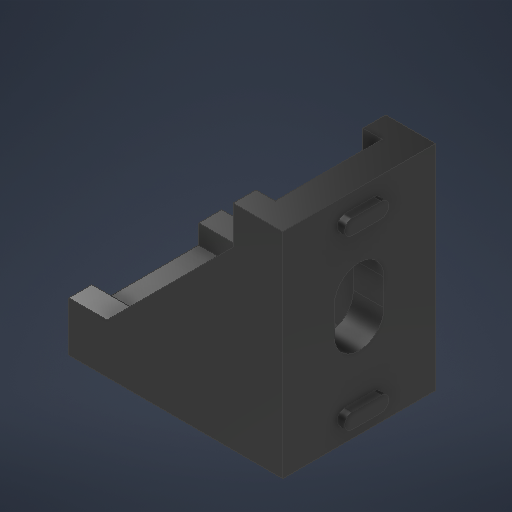
# Autodesk Inventor part: CORNER2028
Saved by Autodesk Inventor 2026.2 (Build 302298010, 298A)
## iProperties
Created: 2026-04-15
Part Number: CORNER2028
Material: Generic
Document SubType Name: Modeling
Designer: grego
Density: 1 g/cm^3
Appearance: Default
Author: grego
Autodesk Inventor part; units mm, degrees
ref_plane "YZ Plane" through (0, 0, 0) normal (1, 0, 0) x (0, 1, 0)
ref_plane "XZ Plane" through (0, 0, 0) normal (0, 1, 0) x (-1, 0, 0)
ref_plane "XY Plane" through (0, 0, 0) normal (0, 0, 1) x (1, 0, 0)
sketch "Sketch1" plane through (0, 0, 0) normal (0, 1, 0) x (-1, 0, 0)
  line L0 (0, 0) -> (28, 0)
  line L1 (28, 0) -> (28, -20)
  line L2 (28, -20) -> (0, -20)
  line L3 (0, -20) -> (0, 0)
  dimension "d0" = 28
  dimension "d1" = 20
  constraints: 8 end point, 2 parallel, 1 horizontal, 1 perpendicular
  measures "d0" distance of L1.end L2.end
  measures "d1" distance of L0.end L1.end
extrude "Extrusion1" add sketch "Sketch1" along normal blind 4
sketch "Sketch2" plane through (0, 4, 0) normal (0, 1, 0) x (1, 0, 0)
  line L0 (0, 20) -> (-28, 20) projected
  line L1 (-28, 20) -> (-28, 0) projected
  line L2 (-28, 0) -> (0, 0) projected
  line L3 (0, 0) -> (0, 20) projected
  line L4 (0, 0) -> (-4, 0)
  line L5 (-4, 0) -> (-4, 20)
  line L6 (-4, 20) -> (0, 20)
  line L7 (0, 20) -> (0, 0)
  dimension "d4" = 4
  constraints: 8 end point, 2 parallel, 1 horizontal, 1 perpendicular, 1 point on line
  measures "d4" distance of L5.end L6.end
extrude "Extrusion2" add sketch "Sketch2" along normal blind 24 contours L3 L2 L5 L0
sketch "Sketch3" plane through (-4, 4, -20) normal (-1, 0, 0) x (0, 0, 1)
  line L0 (20, -4) -> (0, -4) projected
  line L1 (0, -4) -> (0, 24) projected
  line L2 (20, 24) -> (0, 24) projected
  line L3 (20, -4) -> (20, 24) projected
  line L4 (0, -4) -> (0, 24) projected
  line L5 (10, 15.5) -> (10, 15.5)
  line L6 (13.25, 12.25) -> (13.25, 8.75)
  line L7 (10, 5.5) -> (10, 5.5)
  line L8 (6.75, 8.75) -> (6.75, 12.25)
  line L9 (6.75, 15.5) -> (13.25, 5.5) construction
  line L10 (13.25, 15.5) -> (6.75, 5.5) construction
  arc A0 (10, 5.5) -> (13.25, 8.75) centre (10, 8.75) ccw
  arc A1 (6.75, 8.75) -> (10, 5.5) centre (10, 8.75) ccw
  arc A2 (13.25, 12.25) -> (10, 15.5) centre (10, 12.25) ccw
  arc A3 (10, 15.5) -> (6.75, 12.25) centre (10, 12.25) ccw
  point P0 (10, 10.5)
  point P1 (10, 15.5)
  dimension "d7" = 6.5
  dimension "d8" = 10
  dimension "d9" = 3.25
  dimension "d10" = 3.25
  dimension "d11" = 3.25
  constraints: 12 end point, 8 point on circle, 8 point on line, 8 tangent, 4 centre point, 2 midpoint, 2 parallel, 1 concentric, 1 horizontal, 1 perpendicular
  measures "d7" distance of L9.end L10.end
  measures "d8" distance of L10.start L9.end
  measures "d9" radius of A0
  measures "d10" radius of A1
  measures "d11" radius of A2
extrude "Extrusion3" cut sketch "Sketch3" against normal blind 4 contours L6 A0 A1 L8 A3 A2
sketch "Sketch4" plane through (0, 4, 0) normal (0, 1, 0) x (1, 0, 0)
  line L0 (0, 20) -> (-28, 20) projected
  line L1 (0, 0) -> (0, 20) projected
  line L2 (-28, 0) -> (0, 0) projected
  line L3 (-28, 20) -> (-28, 0) projected
  line L4 (-15.75, 6.75) -> (-12.25, 6.75)
  line L5 (-9, 10) -> (-9, 10)
  line L6 (-12.25, 13.25) -> (-15.75, 13.25)
  line L7 (-19, 10) -> (-19, 10)
  line L8 (-19, 6.75) -> (-9, 13.25) construction
  line L9 (-9, 6.75) -> (-19, 13.25) construction
  arc A0 (-9, 10) -> (-12.25, 13.25) centre (-12.25, 10) ccw
  arc A1 (-12.25, 6.75) -> (-9, 10) centre (-12.25, 10) ccw
  arc A2 (-15.75, 13.25) -> (-19, 10) centre (-15.75, 10) ccw
  arc A3 (-19, 10) -> (-15.75, 6.75) centre (-15.75, 10) ccw
  point P0 (-14, 10)
  dimension "d14" = 10
  dimension "d15" = 6.5
  dimension "d16" = 3.25
  constraints: 12 end point, 8 point on circle, 8 point on line, 8 tangent, 4 centre point, 3 equal radius, 2 midpoint, 2 parallel, 1 horizontal, 1 perpendicular
  measures "d14" distance of L9.end L8.end
  measures "d15" distance of L8.end L9.start
  measures "d16" radius of A0
extrude "Extrusion4" cut sketch "Sketch4" against normal blind 4 contours A3 A2 L6 A0 A1 L4
sketch "Sketch5" plane through (0, 0, -20) normal (0, 0, -1) x (-1, 0, 0)
  line L0 (0, 0) -> (28, 0) projected
  line L1 (28, 0) -> (28, 4) projected
  line L2 (4, 4) -> (28, 4) projected
  line L3 (4, 4) -> (4, 28) projected
  line L4 (0, 28) -> (4, 28) projected
  line L5 (0, 0) -> (0, 28) projected
  line L6 (0, 28) -> (6.5, 28)
  line L7 (28, 0) -> (28, 6.5)
  line L8 (28, 6.5) -> (23, 6.5)
  line L9 (6.5, 28) -> (6.5, 23)
  line L10 (6.5, 23) -> (23, 6.5)
  dimension "d19" = 6.5
  dimension "d20" = 6.5
  dimension "d21" = 5
  dimension "d22" = 5
  constraints: 10 end point, 1 horizontal, 1 perpendicular, 1 point on line, 1 vertical
  measures "d19" distance of L4.start L6.end
  measures "d20" distance of L0.end L7.end
  measures "d21" distance of L7.end L8.end
  measures "d22" distance of L6.end L9.end
extrude "Extrusion5" add sketch "Sketch5" against normal blind 3 contours L2 L3 L6 L9 L10 L8 L7
sketch "Sketch6" plane through (-28, 0, 0) normal (0, 0, 1) x (1, 0, 0)
  line L0 (21.5, 23) -> (5, 6.5) projected
  line L1 (5, 6.5) -> (0, 6.5) projected
  line L2 (0, 6.5) -> (0, 4) projected
  line L3 (24, 4) -> (0, 4) projected
  line L4 (24, 28) -> (24, 4) projected
  line L5 (24, 28) -> (21.5, 28) projected
  line L6 (21.5, 28) -> (21.5, 23) projected
  line L7 (0, 0) -> (28, 0) projected
  line L8 (28, 0) -> (28, 28) projected
  line L9 (24, 28) -> (28, 28) projected
  line L10 (24, 4) -> (24, 28) projected
  line L11 (0, 4) -> (24, 4) projected
  line L12 (0, 0) -> (0, 4) projected
extrude "Extrusion6" add sketch "Sketch6" against normal blind 3 contours L6 L5 L4 L3 L2 L1 L0
sketch "Sketch7" plane through (0, 0, 0) normal (1, 0, 0) x (0, 0, -1)
  line L0 (3, 4) -> (17, 4) projected
  line L1 (10, 4) -> (10, 3)
  line L2 (8.1, 2) -> (11.9, 2)
  line L3 (12.9, 3) -> (12.9, 3)
  line L4 (11.9, 4) -> (8.1, 4)
  line L5 (7.1, 3) -> (7.1, 3)
  line L6 (7.1, 2) -> (12.9, 4) construction
  line L7 (12.9, 2) -> (7.1, 4) construction
  arc A0 (8.1, 4) -> (7.1, 3) centre (8.1, 3) ccw
  arc A1 (7.1, 3) -> (8.1, 2) centre (8.1, 3) ccw
  arc A2 (12.9, 3) -> (11.9, 4) centre (11.9, 3) ccw
  arc A3 (11.9, 2) -> (12.9, 3) centre (11.9, 3) ccw
  point P0 (0, 0)
  dimension "d27" = 1
  dimension "d28" = 5.8
  dimension "d29" = 1
  constraints: 14 end point, 9 point on line, 8 point on circle, 8 tangent, 4 centre point, 3 equal radius, 3 midpoint, 2 parallel, 1 horizontal, 1 perpendicular, 1 vertical
  measures "d27" distance of L1.start L1.end
  measures "d28" distance of L7.end L6.end
  measures "d29" radius of A0
extrude "Extrusion7" add sketch "Sketch7" along normal blind 1
sketch "Sketch8" plane through (0, 0, 0) normal (0, -1, 0) x (1, 0, 0)
  line L0 (-4, -3) -> (-4, -17) projected
  line L1 (-4, -10) -> (-3, -10)
  line L2 (-3, -7.1) -> (-3, -7.1)
  line L3 (-4, -8.1) -> (-4, -11.9)
  line L4 (-3, -12.9) -> (-3, -12.9)
  line L5 (-2, -11.9) -> (-2, -8.1)
  line L6 (-2, -7.1) -> (-4, -12.9) construction
  line L7 (-4, -7.1) -> (-2, -12.9) construction
  arc A0 (-4, -11.9) -> (-3, -12.9) centre (-3, -11.9) ccw
  arc A1 (-3, -12.9) -> (-2, -11.9) centre (-3, -11.9) ccw
  arc A2 (-2, -8.1) -> (-3, -7.1) centre (-3, -8.1) ccw
  arc A3 (-3, -7.1) -> (-4, -8.1) centre (-3, -8.1) ccw
  point P0 (0, 0)
  dimension "d32" = 1
  dimension "d33" = 5.8
  dimension "d34" = 1
  constraints: 14 end point, 9 point on line, 8 point on circle, 8 tangent, 4 centre point, 3 equal radius, 3 midpoint, 2 horizontal, 2 parallel, 1 perpendicular
  measures "d32" distance of L1.start L1.end
  measures "d33" distance of L6.end L7.start
  measures "d34" radius of A0
extrude "Extrusion8" add sketch "Sketch8" along normal blind 1
sketch "Sketch9" plane through (0, 0, 0) normal (0, -1, 0) x (1, 0, 0)
  line L0 (-28, -20) -> (-28, 0) projected
  line L1 (-28, -10) -> (-25, -10)
  line L2 (-25, -12.9) -> (-25, -12.9)
  line L3 (-26, -11.9) -> (-26, -8.1)
  line L4 (-25, -7.1) -> (-25, -7.1)
  line L5 (-24, -8.1) -> (-24, -11.9)
  line L6 (-24, -12.9) -> (-26, -7.1) construction
  line L7 (-26, -12.9) -> (-24, -7.1) construction
  arc A0 (-26, -11.9) -> (-25, -12.9) centre (-25, -11.9) ccw
  arc A1 (-25, -7.1) -> (-26, -8.1) centre (-25, -8.1) ccw
  arc A2 (-24, -8.1) -> (-25, -7.1) centre (-25, -8.1) ccw
  arc A3 (-25, -12.9) -> (-24, -11.9) centre (-25, -11.9) ccw
  point P0 (0, 0)
  dimension "d37" = 3
  dimension "d38" = 2
  dimension "d39" = 5.8
  dimension "d40" = 1
  constraints: 14 end point, 8 point on circle, 8 point on line, 8 tangent, 4 centre point, 3 equal radius, 3 midpoint, 2 horizontal, 2 parallel, 1 perpendicular
  measures "d37" distance of L1.start L1.end
  measures "d38" distance of L6.end L7.end
  measures "d39" distance of L7.start L6.end
  measures "d40" radius of A0
extrude "Extrusion9" add sketch "Sketch9" along normal blind 1
sketch "Sketch10" plane through (0, 0, 0) normal (1, 0, 0) x (0, 0, -1)
  line L0 (17, 28) -> (3, 28) projected
  line L1 (10, 28) -> (10, 25)
  line L2 (8.1, 24) -> (11.9, 24)
  line L3 (12.9, 25) -> (12.9, 25)
  line L4 (11.9, 26) -> (8.1, 26)
  line L5 (7.1, 25) -> (7.1, 25)
  line L6 (7.1, 24) -> (12.9, 26) construction
  line L7 (12.9, 24) -> (7.1, 26) construction
  arc A0 (8.1, 26) -> (7.1, 25) centre (8.1, 25) ccw
  arc A1 (12.9, 25) -> (11.9, 26) centre (11.9, 25) ccw
  arc A2 (11.9, 24) -> (12.9, 25) centre (11.9, 25) ccw
  arc A3 (7.1, 25) -> (8.1, 24) centre (8.1, 25) ccw
  point P0 (0, 0)
  dimension "d43" = 3
  dimension "d44" = 5.8
  dimension "d45" = 2
  dimension "d46" = 1
  constraints: 14 end point, 8 point on circle, 8 point on line, 8 tangent, 4 centre point, 3 equal radius, 3 midpoint, 2 parallel, 1 horizontal, 1 perpendicular, 1 vertical
  measures "d43" distance of L1.start L1.end
  measures "d44" distance of L7.end L6.end
  measures "d45" distance of L6.end L7.start
  measures "d46" radius of A0
extrude "Extrusion10" add sketch "Sketch10" along normal blind 1
body "Solid1"
